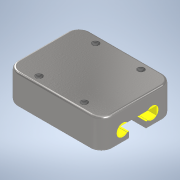
# Autodesk Inventor part: Fuehrungslager
Saved by Autodesk Inventor 2021.3 (Build 253353000, 353)
## iProperties
Created: 2021-04-14
Part Number: Fuehrungslager
Material: Generic
Document SubType Name: Modeling
Designer: Fabijan_Sven
Density: 1 g/cm^3
Appearance: Smooth - Yellow
Author: Fabijan_Sven
Autodesk Inventor part; units mm, degrees
ref_plane "YZ Plane" through (0, 0, 0) normal (1, 0, 0) x (0, 1, 0)
ref_plane "XZ Plane" through (0, 0, 0) normal (0, 1, 0) x (-1, 0, 0)
ref_plane "XY Plane" through (0, 0, 0) normal (0, 0, 1) x (1, 0, 0)
sketch "Sketch1" plane through (0, 0, 0) normal (1, 0, 0) x (0, 1, 0)
  line L0 (0, 0) -> (13.2, 0)
  line L1 (13.2, 0) -> (13.2, -32)
  line L2 (13.2, -32) -> (0, -32)
  line L3 (0, -32) -> (0, -19.7414)
  arc A0 (7, -11.5) -> (3.2, -11.5) centre (5.1, -9.5) ccw
  arc A1 (3.2, -20.5) -> (7, -20.5) centre (5.1, -22.5) ccw
  line L4 (3.2, -11.5) -> (3.2, -12.2586)
  line L5 (0, -12.2586) -> (0, 0)
  line L6 (7, -20.5) -> (7, -11.5)
  line L7 (3.2, -19.7414) -> (3.2, -20.5)
  line L8 (3.2, -19.7414) -> (0, -19.7414)
  line L9 (0, -12.2586) -> (3.2, -12.2586)
  dimension "d0" = 32
  dimension "d1" = 13.2
  dimension "d9" = 9.5
  dimension "d10" = 9.5
  dimension "d11" = 2.7586
  dimension "d12" = 2.7586
  dimension "d13" = 7
  dimension "d14" = 3.2
  dimension "d15" = 5.1
  dimension "d16" = 5.1
  dimension "d17" = 0.7586
  dimension "d18" = 0.7586
  dimension "d19" = 9
  dimension "d20" = 3.2
  constraints: 20 end point, 6 parallel, 4 point on circle, 2 centre point, 2 horizontal, 1 perpendicular
  measures "d0" distance of L0.end L1.end
  measures "d1" distance of L1.end L2.end
  measures "d9" distance from line of L0 A0.centre
  measures "d10" distance from line of L2 A1.centre
  measures "d11" radius of A1
  measures "d12" radius of A0
  measures "d13" distance between parallel lines of L3 L6
  measures "d14" distance between parallel lines of L3 L7
  measures "d15" distance from line of L3 A1.centre
  measures "d16" distance from line of L5 A0.centre
  measures "d17" distance of L4.start L4.end
  measures "d18" distance of L7.start L7.end
  measures "d19" distance of L6.end L6.start
  measures "d20" distance of L5.start L4.end
extrude "Extrusion1" add sketch "Sketch1" along normal blind 42
sketch "Sketch2" plane through (0, 13.2, 0) normal (0, 1, 0) x (1, 0, 0)
  circle A0 centre (11, 3.5) radius 1.5
  circle A1 centre (31, 3.5) radius 1.4957
  line L0 (-3.7091, 16) -> (49.3641, 16) construction
  line L1 (0, 0) -> (42, 0) projected
  circle A2 centre (11, 28.5) radius 1.5
  circle A3 centre (31, 28.5) radius 1.4957
  line L2 (0, 32) -> (0, 0) projected
  dimension "d23" = 16
  dimension "d24" = 3
  dimension "d25" = 20
  dimension "d26" = 11
  dimension "d27" = 3.5
  dimension "d28" = 3.5
  constraints: 4 centre point, 2 end point, 2 symmetric about line, 1 horizontal, 2 other
  measures "d23" distance between parallel lines of L1 L0
  measures "d24" diameter of A0
  measures "d25" distance of A1.centre A0.centre
  measures "d26" distance from line of L2 A0.centre
  measures "d27" distance from line of L1 A0.centre
  measures "d28" distance from line of L1 A1.centre
extrude "Extrusion2" cut sketch "Sketch2" against normal blind 10
sketch "Sketch3" plane through (42, 0, 0) normal (1, 0, 0) x (0, 0, -1)
  arc A0 (11.5, 7) -> (7.5817, 7.0824) centre (9.5, 5.1) ccw
  arc A1 (20.5, 3.2) -> (24.5, 3.2) centre (22.5, 5.1) ccw
  arc A2 (11.5, 7) -> (11.5, 3.2) centre (9.5, 5.1) ccw projected
  arc A3 (20.5, 3.2) -> (20.5, 7) centre (22.5, 5.1) ccw projected
  line L0 (11.5, 7) -> (20.5, 7) projected
  line L1 (11.5, 7) -> (20.5, 7)
  line L2 (7.5817, 7) -> (24.4183, 7)
  line L3 (24.4183, 7) -> (24.4183, 3.2)
  line L4 (24.4183, 3.2) -> (20.5, 3.2)
  line L5 (7.5817, 3.2) -> (7.5817, 7)
  arc A4 (7.5, 3.2) -> (11.5, 3.2) centre (9.5, 5.1) ccw
  arc A5 (7.5817, 7.0824) -> (7.5, 7) centre (9.5, 5.1) ccw
  arc A6 (7.5, 7) -> (7.5, 3.2) centre (9.5, 5.1) ccw
  arc A7 (24.5, 7) -> (24.4183, 7.0824) centre (22.5, 5.1) ccw
  arc A8 (24.5, 3.2) -> (24.5, 7) centre (22.5, 5.1) ccw
  arc A9 (24.4183, 7.0824) -> (20.5, 7) centre (22.5, 5.1) ccw
  line L6 (11.5, 3.2) -> (7.5817, 3.2)
  arc A10 (20.5817, 3.2) -> (20.5817, 7) centre (22.5, 5.1) ccw
  arc A11 (11.4183, 7) -> (11.4183, 3.2) centre (9.5, 5.1) ccw
  point P0 (0, 0)
  dimension "d31" = 3.8
  dimension "d32" = 5.4
  dimension "d33" = 5.4
  constraints: 24 point on circle, 12 end point, 10 centre point, 8 point on line, 4 concentric, 3 parallel, 2 coincident, 2 horizontal, 1 perpendicular
  measures "d31" distance of L5.start L2.start
  measures "d32" diameter of A10
  measures "d33" diameter of A11
extrude "Extrusion3" add sketch "Sketch3" against normal up to surface (42 mm away) contours L2 A11 | A10 L2 | L5 A11 | A10 L3 | L6 A11 | A10 L4
fillet "Fillet1" radius 5 4 edges at (0, 6.6, 0) (0, 6.6, -32) (42, 6.6, 0) (42, 6.6, -32)
fillet "Fillet2" radius 1 20 edges at (40.5355, 13.2, -30.5355) (42, 13.2, -16) (40.5355, 13.2, -1.4645) (21, 13.2, 0) (1.4645, 13.2, -1.4645) (0, 13.2, -16) (1.4645, 13.2, -30.5355) (21, 13.2, -32) (40.5355, 0, -30.5355) (42, 0, -23.3707) (1.4645, 0, -30.5355) (0, 0, -23.3707) (21, 0, -32) (40.5355, 0, -1.4645) (42, 0, -8.6293) (1.4645, 0, -1.4645) (0, 0, -8.6293) (21, 0, 0) (21, 0, -12.2586) (21, 0, -19.7414)
thread "Thread1" size "M3x0.5" class "6H" standard "ISO Metric profile" full length
thread "Thread2" size "M3x0.5" class "6H" standard "ISO Metric profile" full length
thread "Thread3" size "M3x0.5" class "6H" standard "ISO Metric profile" full length
thread "Thread4" size "M3x0.5" class "6H" standard "ISO Metric profile" full length
body "Solid1"
